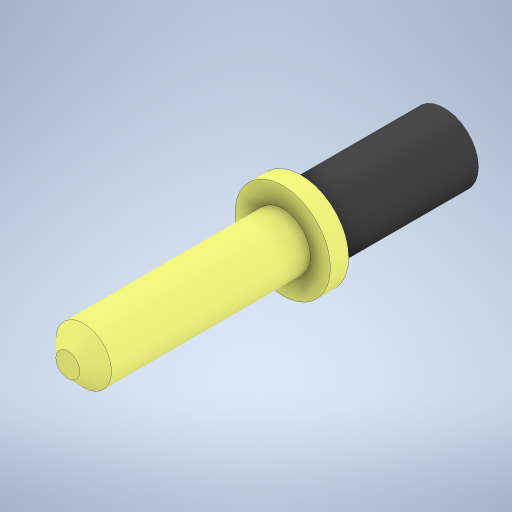
# Autodesk Inventor part: Audio_jac
Saved by Autodesk Inventor 2023.1 (Build 271208000, 208)
## iProperties
Created: 2022-08-09
Part Number: Audio_jac
Material: 일반
Document SubType Name: Modeling
Designer: fly01
Density: 1 g/cm^3
Appearance: 기본값
Author: fly01
Autodesk Inventor part; units mm, degrees
ref_plane "YZ Plane" through (0, 0, 0) normal (1, 0, 0) x (0, 1, 0)
ref_plane "XZ Plane" through (0, 0, 0) normal (0, 1, 0) x (-1, 0, 0)
ref_plane "XY Plane" through (0, 0, 0) normal (0, 0, 1) x (1, 0, 0)
sketch "스케치1" plane through (0, 0, 0) normal (0, 0, 1) x (1, 0, 0)
  circle A0 centre (0, 0) radius 1.75
  circle A1 centre (0, 0) radius 3
  circle A2 centre (0, 0) radius 2.15
  dimension "d0" = 3.5
  dimension "d1" = 6
  dimension "d2" = 4.3
  constraints: 3 centre point, 3 coincident
  measures "d0" diameter of A0
  measures "d1" diameter of A1
  measures "d2" diameter of A2
extrude "돌출1" add sketch "스케치1" along normal blind 13.5 contours A0
extrude "돌출2" add sketch "스케치1" against normal blind 1.15 contours A0 | A1 | A2
extrude "돌출3" add sketch "스케치1" against normal blind 10.15 contours A0 | A2
chamfer "모따기1" distance 1 angle 45 1 edges at (-1.75, 0, 13.5)
